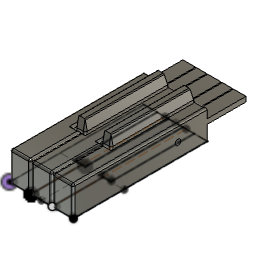
PianoKeys v7 (Autodesk Fusion 360 design; units mm, degrees)
Autodesk Fusion 360 part; units mm, degrees
note: some values were not read from the file. Chosen so that the rebuilt part matches the saved one: which pieces of a blend or face edit are solid.
sketch "Sketch2" plane through (0, 0, 0) normal (0, 0, 1) x (1, 0, 0)
  line L0 (0, 0) -> (19.5, 0) construction
  line L1 (0, 0) -> (0, 138) construction
  line L2 (0, 138) -> (22, 138) construction
  line L3 (22, 138) -> (22, 0) construction
  line L4 (22, 138) -> (22, 0) construction
  line L5 (0, 0) -> (0.5, 0) construction
  line L6 (0.5, 2) -> (0.5, 138)
  line L7 (2.5, 0) -> (21.5, 0)
  line L8 (21.5, 2) -> (21.5, 52)
  line L9 (0, 138) -> (13.92, 138) construction
  line L10 (13.92, 138) -> (25.42, 138) construction
  line L11 (25.42, 138) -> (25.42, 53) construction
  line L12 (25.42, 53) -> (16.42, 53) construction
  line L13 (13.92, 53) -> (13.92, 138) construction
  line L14 (21.5, 52) -> (0, 52) construction
  line L15 (0, 138) -> (13.42, 138) construction
  line L16 (13.42, 138) -> (13.42, 52)
  line L17 (21.5, 52) -> (13.42, 52)
  line L18 (13.42, 138) -> (0.5, 138)
  line L19 (13.92, 138) -> (14.42, 138) construction
  line L20 (14.42, 138) -> (24.92, 138)
  line L21 (24.92, 138) -> (24.92, 55)
  line L22 (22.92, 53) -> (14.42, 53)
  line L23 (14.42, 55) -> (14.42, 138)
  line L24 (22.5, 2) -> (22.5, 52)
  line L25 (44, 138) -> (22, 138) construction
  line L26 (43.5, 138) -> (25.92, 138) construction
  line L27 (25.92, 138) -> (25.92, 52) construction
  line L28 (44, 0) -> (22, 0) construction
  line L29 (25.92, 138) -> (33, 138)
  line L30 (22.5, 52) -> (25.92, 52)
  line L31 (25.92, 138) -> (25.92, 52)
  line L32 (24.5, 0) -> (33, 0)
  line L33 (33, 138) -> (33, 0) construction
  arc A0 (0.5, 2) -> (2.5, 0) centre (2.5, 2) ccw
  arc A1 (19.5, 0) -> (21.5, 2) centre (19.5, 2) ccw
  arc A2 (22.5, 2) -> (24.5, 0) centre (24.5, 2) ccw
  arc A3 (14.42, 55) -> (16.42, 53) centre (16.42, 55) ccw
  arc A4 (22.92, 53) -> (24.92, 55) centre (22.92, 55) ccw
  arc A5 (41.08, 55) -> (43.08, 53) centre (43.08, 55) ccw
  line L34 (43.5, 52) -> (40.08, 52)
  line L35 (43.08, 53) -> (51.58, 53)
  line L36 (44.5, 52) -> (66, 52) construction
  arc A6 (49.58, 53) -> (51.58, 55) centre (49.58, 55) ccw
  arc A7 (63.5, 0) -> (65.5, 2) centre (63.5, 2) ccw
  line L37 (40.58, 53) -> (49.58, 53) construction
  line L38 (40.58, 138) -> (40.58, 53) construction
  line L39 (40.08, 138) -> (40.08, 52) construction
  line L40 (52.58, 138) -> (52.58, 52)
  line L41 (66, 138) -> (52.58, 138) construction
  line L42 (22, 0) -> (44, 0) construction
  arc A8 (44.5, 2) -> (46.5, 0) centre (46.5, 2) ccw
  line L43 (40.08, 138) -> (33, 138)
  arc A9 (41.5, 0) -> (43.5, 2) centre (41.5, 2) ccw
  line L44 (41.5, 0) -> (33, 0)
  line L45 (52.08, 53) -> (52.08, 138) construction
  line L46 (52.08, 138) -> (51.58, 138) construction
  line L47 (63.5, 0) -> (44.5, 0)
  line L48 (40.08, 138) -> (40.08, 52)
  line L49 (52.08, 138) -> (40.58, 138) construction
  line L50 (66, 0) -> (65.5, 0) construction
  line L51 (66, 0) -> (46.5, 0) construction
  line L52 (51.58, 55) -> (51.58, 138)
  line L53 (44.5, 2) -> (44.5, 52)
  line L54 (44.5, 52) -> (52.58, 52)
  line L55 (44, 138) -> (44, 0) construction
  line L56 (41.08, 138) -> (41.08, 55)
  line L57 (52.58, 138) -> (65.5, 138)
  line L58 (66, 138) -> (44, 138) construction
  line L59 (43.5, 2) -> (43.5, 52)
  line L60 (44, 138) -> (44, 0) construction
  line L61 (66, 0) -> (66, 138) construction
  line L62 (22.5, 138) -> (40.08, 138) construction
  line L63 (66, 138) -> (52.08, 138) construction
  line L64 (51.58, 138) -> (41.08, 138)
  line L65 (65.5, 2) -> (65.5, 138)
  line L66 (22, 138) -> (44, 138) construction
  point P0 (24.92, 53)
  point P1 (22.5, 0)
  point P2 (41.08, 53)
  point P3 (43.5, 0)
  point P4 (66, 0)
  dimension "d14" = 138
  dimension "d15" = 22
  dimension "d16" = 22
  dimension "d25" = 138
  dimension "d26" = 21
  dimension "d27" = 52
  dimension "d29" = 13.92
  dimension "d30" = 11.5
  dimension "d31" = 85
  dimension "d32" = 13.42
  dimension "d33" = 0.5
  dimension "d34" = 85
  dimension "d35" = 10.5
  dimension "d36" = 0.5
  dimension "d37" = 22
  dimension "d38" = 17.58
  dimension "d39" = 86
  dimension "d40" = 7.08
  dimension "d41" = 10.5
  dimension "d43" = 2
  dimension "d44" = 2
  dimension "d45" = 2
  dimension "d48" = 2
  constraint coincident L0.start L1.start
  constraint horizontal L0
  constraint perpendicular L0 L1
  constraint perpendicular L1 L2
  constraint perpendicular L1 L5
  constraint perpendicular L2 L6
  constraint perpendicular L6 L7
  constraint perpendicular L0 L8
  constraint perpendicular L1 L9
  constraint horizontal L10
  constraint vertical L11
  constraint horizontal L12
  constraint vertical L13
  constraint coincident L1 L14.end
  constraint perpendicular L1 L14
  constraint perpendicular L1 L15
  constraint coincident L14 L16.end
  constraint perpendicular L14 L16
  constraint perpendicular L13 L19
  constraint horizontal L20
  constraint vertical L21
  constraint horizontal L22
  constraint vertical L23
  constraint symmetric L1.end L3 L25.start
  constraint symmetric L3 L6.end L26.start
  constraint symmetric L3 L7.end P1
  constraint symmetric L3 L8.end L24.end
  constraint perpendicular L3 L25
  constraint perpendicular L25 L27
  constraint symmetric L0.start L3 L28.start
  constraint symmetric L4.end L3 L28.end
  constraint perpendicular L27 L29
  constraint perpendicular L27 L30
  constraint perpendicular L24 L32
  constraint coincident L5.end L6
  constraint coincident L5.end L7
  constraint tangent L6 A0
  constraint tangent L7 A0
  constraint coincident L7.end L8
  constraint coincident L3.end L0
  constraint tangent L8 A1
  constraint tangent L0 A1
  constraint coincident P1 L32
  constraint coincident P1 L24
  constraint tangent L32 A2
  constraint tangent L24 A2
  constraint coincident L13.start L12
  constraint coincident L22.end L23
  constraint tangent L12 A3
  constraint tangent L23 A3
  constraint coincident P0 L21
  constraint coincident P0 L22
  constraint tangent L21 A4
  constraint tangent L22 A4
  constraint equal A3 A4
  constraint symmetric L0.start L33 P4
  constraint symmetric L3.end L33 L28.start
  constraint symmetric L1.end L33 L41.start
  constraint symmetric L2.end L33 L25.start
  constraint symmetric L5.end L33 L50.end
  constraint symmetric L6.end L33 L57.end
  constraint symmetric L7.end L33 L47.end
  constraint symmetric L8.end L33 L36.start
  constraint symmetric L9.end L33 L45.end
  constraint symmetric L10.end L33 L38.start
  constraint symmetric L11.end L33 L37.start
  constraint symmetric L13.start L33 L45.start
  constraint symmetric L14.end L33 L36.end
  constraint symmetric L15.end L33 L40.start
  constraint symmetric L16.end L33 L40.end
  constraint symmetric L19.end L33 L46.end
  constraint symmetric L20.end L33 L56.start
  constraint symmetric P0 L33 P2
  constraint symmetric L22.end L33 L35.end
  constraint symmetric L26.start L33 L62.start
  constraint symmetric L25.start L33 L2.end
  constraint symmetric P1 L33 P3
  constraint symmetric L24.end L33 L34.start
  constraint symmetric L26.end L33 L39.start
  constraint symmetric L27.end L33 L34.end
  constraint symmetric L28.start L33 L3.end
  constraint symmetric L29.end L33 L43.end
  constraint symmetric L32.end L33 L44.end
  constraint symmetric L33 L6.start A7.end
  constraint symmetric L33 L7.start A7.start
  constraint symmetric L33 A0 A7
  constraint symmetric L33 L8.start A8.start
  constraint symmetric L33 L0.end A8.end
  constraint symmetric L33 A1 A8
  constraint symmetric L33 L32.start A9.start
  constraint symmetric L33 L24.start A9.end
  constraint symmetric L33 A2 A9
  constraint symmetric L33 L12.end A6.start
  constraint symmetric L33 L23.start A6.end
  constraint symmetric L33 A3 A6
  constraint symmetric L33 L21.end A5.start
  constraint symmetric L33 L22.start A5.end
  constraint symmetric L33 A4 A5
  measures "d14" distance of L0.start L1.end
  measures "d15" distance of L0.start L3.end
  measures "d16" distance of L1.end L2.end
  measures "d25" distance of L5.end L6.end
  measures "d26" distance of L5.end L7.end
  measures "d27" distance of L7.end L8.end
  measures "d29" distance of L1.end L9.end
  measures "d30" distance of L11.end L13.start
  measures "d31" distance of L10.end L11.end
  measures "d32" distance of L1.end L15.end
  measures "d33" distance of L9.end L19.end
  measures "d34" distance of L20.end P0
  measures "d35" distance of L19.end L20.end
  measures "d36" distance of L0.start L5.end
  measures "d37" distance of L2.end L25.start
  measures "d38" distance of L26.start L26.end
  measures "d39" distance of L26.end L27.end
  measures "d40" distance of L26.end L29.end
  measures "d41" distance of P1 L32.end
  measures "d43" radius of A0
  measures "d44" radius of A1
  measures "d45" radius of A2
  measures "d48" radius of A3
extrude "Extrude1" add sketch "Sketch2" along normal blind 30 contours L6 L7 L8 L16 L17 L18 A0 A1 | L24 L29 L30 L31 L32 A2 L34 L43 A9 L44 L48 L59 | A7 L40 A8 L47 L53 L54 L57 L65 makes body 1 at (0.5, 47.3333, 10) makes body 2 at (25.92, 109.3333, 10) makes body 3 at (65.5, 47.3333, 10)
extrude "Extrude2" add sketch "Sketch2" along normal blind 40 separate body contours L20 L21 L22 L23 A3 A4 | A5 L35 A6 L52 L56 L64 makes body 4 at (24.92, 110.3333, 13.3333) makes body 5 at (41.08, 82.6667, 13.3333)
chamfer "Chamfer1" distance 2 distance2 10 2 faces at (17.92, 110.3333, 40) (44.58, 110.3333, 40) on bodies 4 5
fillet "Fillet1" radius 2 3 faces at (11.8067, 18.6667, 30) (30.64, 18.6667, 30) (54.1933, 18.6667, 30) on bodies 1 2 3
sketch "Sketch3" plane through (0.5, 0, 0) normal (-1, 0, 0) x (0, -1, 0)
  line L0 (-2, 28) -> (-138, 28)
  line L1 (-138, 28) -> (-138, 0)
  line L2 (-138, 0) -> (-2, 0)
  line L3 (-2, 0) -> (-2, 28)
  line L4 (-138, 0) -> (-138, 14) construction
  line L5 (-138, 14) -> (-108, 14) construction
  circle A0 centre (-108, 14) radius 2.9
  dimension "d62" = 30
  dimension "d63" = 5.8
  constraint coincident L1.end L2.start
  constraint midpoint L1 L4.end
  constraint perpendicular L4 L5
  constraint coincident L5.end A0.centre
  measures "d62" distance of L4.end L5.end
  measures "d63" diameter of A0
extrude "Extrude3" cut sketch "Sketch3" against normal blind 10000 contours A0 bodies 1 2 3 4 5
fillet "Fillet2" radius 1 4 edges at (16.42, 95.5, 40) (22.92, 95.5, 40) (43.08, 95.5, 40) (49.58, 95.5, 40) on bodies 4 5
sketch "Sketch4" plane through (0, 0, 0) normal (0, 0, 1) x (1, 0, 0)
sketch "Sketch11" plane through (0, 138, 0) normal (0, 1, 0) x (-1, 0, 0)
  line L0 (-0.5, 28) -> (-13.42, 28)
  line L1 (-13.42, 28) -> (-13.42, 0)
  line L2 (-13.42, 0) -> (-0.5, 0)
  line L3 (-0.5, 0) -> (-0.5, 28)
  line L4 (-0.5, 0) -> (-0.5, 15) construction
  line L5 (-0.5, 15) -> (-13.42, 15)
  line L6 (-13.42, 15) -> (-13.42, 20)
  line L7 (-13.42, 20) -> (-0.5, 20)
  line L8 (-0.5, 20) -> (-0.5, 15)
  line L9 (-0.5, 15) -> (-96.3379, 15) construction
  line L10 (-0.5, 20) -> (-96.473, 20) construction
  line L11 (-0.5, 15) -> (-14.42, 15) construction
  line L12 (-14.42, 15) -> (-24.92, 15)
  line L13 (-24.92, 15) -> (-24.92, 20)
  line L14 (-24.92, 20) -> (-14.42, 20)
  line L15 (-14.42, 20) -> (-14.42, 15)
  line L16 (-33, 0) -> (-33, 28) construction
  line L17 (-24.92, 15) -> (-25.92, 15) construction
  line L18 (-25.92, 15) -> (-33, 15) construction
  line L19 (-33, 15) -> (-33, 20) construction
  line L20 (-33, 20) -> (-25.92, 20) construction
  line L21 (-25.92, 20) -> (-25.92, 15) construction
  line L22 (-25.92, 15) -> (-33, 15)
  line L23 (-33, 20) -> (-25.92, 20)
  line L24 (-25.92, 20) -> (-25.92, 15)
  line L25 (-40.08, 15) -> (-33, 15) construction
  line L26 (-51.58, 15) -> (-41.08, 15)
  line L27 (-40.08, 20) -> (-40.08, 15)
  line L28 (-41.08, 20) -> (-51.58, 20)
  line L29 (-41.08, 15) -> (-40.08, 15) construction
  line L30 (-40.08, 20) -> (-40.08, 15) construction
  line L31 (-40.08, 15) -> (-33, 15)
  line L32 (-52.58, 20) -> (-65.5, 20)
  line L33 (-41.08, 15) -> (-41.08, 20)
  line L34 (-65.5, 15) -> (-52.58, 15)
  line L35 (-52.58, 15) -> (-52.58, 20)
  line L36 (-51.58, 20) -> (-51.58, 15)
  line L37 (-33, 15) -> (-33, 20)
  line L38 (-33, 20) -> (-40.08, 20)
  line L39 (-65.5, 20) -> (-65.5, 15)
  line L40 (-65.5, 15) -> (-51.58, 15) construction
  line L41 (-33, 20) -> (-40.08, 20) construction
  dimension "d70" = 15
  dimension "d71" = 12.92
  dimension "d72" = 5
  dimension "d73" = 13.92
  dimension "d74" = 10.5
  dimension "d75" = 5
  dimension "d76" = 1
  constraint coincident L2.end L3.start
  constraint perpendicular L2 L4
  constraint horizontal L5
  constraint vertical L6
  constraint horizontal L7
  constraint vertical L8
  constraint perpendicular L4 L9
  constraint perpendicular L8 L10
  constraint coincident L9 L11.end
  constraint horizontal L12
  constraint vertical L13
  constraint horizontal L14
  constraint vertical L15
  constraint perpendicular L2 L16
  constraint perpendicular L13 L17
  constraint horizontal L18
  constraint vertical L19
  constraint horizontal L20
  constraint vertical L21
  constraint coincident L10 L19.end
  constraint coincident L16 L19.end
  constraint horizontal L22
  constraint horizontal L23
  constraint vertical L24
  constraint symmetric L4.end L16 L34.start
  constraint symmetric L5.end L16 L34.end
  constraint symmetric L6.end L16 L32.start
  constraint symmetric L7.end L16 L32.end
  constraint symmetric L11.end L16 L26.start
  constraint symmetric L12.end L16 L26.end
  constraint symmetric L13.end L16 L28.start
  constraint symmetric L14.end L16 L28.end
  constraint symmetric L16 L17.end L25.start
  constraint symmetric L16 L18.end L19.start
  constraint symmetric L16 L19.end L20.start
  constraint symmetric L16 L20.end L27.start
  measures "d70" distance of L2.end L4.end
  measures "d71" distance of L4.end L5.end
  measures "d72" distance of L4.end L7.end
  measures "d73" distance of L4.end L11.end
  measures "d74" distance of L11.end L12.end
  measures "d75" distance of L11.end L14.end
  measures "d76" distance of L12.end L17.end
extrude "Extrude4" add sketch "Sketch11" along normal blind 40 contours L1 L3 L5 L6 L7 L8 | L12 L13 L14 L15 | L22 L23 L24 L37 | L27 L31 L37 L38 | L26 L28 L33 L36 | L32 L34 L35 L39 bodies 1 2 3 4 5
equation "WhiteKeyLength = 138 mm"
equation "WhiteKeyWidth = 22 mm"
equation "BlackKeyWidth = 11.5 mm"
equation "BlackKeyLength = 85 mm"
equation "Cdisplacement = 13.92 mm"
equation "buffer = 0.5 mm"
equation "d14 = WhiteKeyLength"
equation "d15 = WhiteKeyWidth"
equation "d16 = WhiteKeyWidth"
equation "d25 = WhiteKeyLength"
equation "d26 = WhiteKeyWidth - 2 * buffer"
equation "d27 = WhiteKeyLength - BlackKeyLength - VerticalBuffer"
equation "blackKeyOffset = 13.92 mm"
equation "d29 = blackKeyOffset"
equation "d30 = BlackKeyWidth"
equation "d31 = BlackKeyLength"
equation "d32 = blackKeyOffset - buffer"
equation "d33 = buffer"
equation "d34 = BlackKeyLength"
equation "d35 = BlackKeyWidth - 2 * buffer"
equation "d36 = buffer"
equation "d37 = WhiteKeyWidth"
equation "d38 = 2 * WhiteKeyWidth - blackKeyOffset - BlackKeyWidth - 2 * buffer"
equation "d39 = BlackKeyLength + VerticalBuffer"
equation "d40 = 2 * WhiteKeyWidth - blackKeyOffset - BlackKeyWidth - 2 * buffer - 0.5 * ( WhiteKeyWidth - 2 * buffer )"
equation "d41 = 0.5 * ( WhiteKeyWidth - 2 * buffer )"
equation "filletDepth = 2 mm"
equation "d43 = filletDepth"
equation "d44 = filletDepth"
equation "d45 = filletDepth"
equation "d48 = filletDepth"
equation "whiteKeyHeight = 30 mm"
equation "d51 = whiteKeyHeight"
equation "blackKeyHeight = 40 mm"
equation "d54 = blackKeyHeight"
equation "VerticalBuffer = 1 mm"
equation "HoleDistance = 30 mm"
equation "d62 = HoleDistance"
equation "d70 = whiteKeyHeight / 2"
equation "d71 = blackKeyOffset - 2 * buffer"
equation "d73 = blackKeyOffset"
equation "d74 = BlackKeyWidth - 2 * buffer"
equation "d76 = 2 * buffer"
